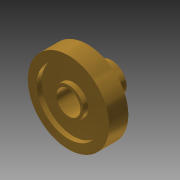
# Autodesk Inventor part: Spur Gear
Saved by Autodesk Inventor 2015 SP1 (Build 190203100, 203)
## iProperties
Created: 2015-02-24
Part Number: Spur Gear
Material: Brass, Soft Yellow
Document SubType Name: Modeling
Designer: Andrew
Density: 8.47 g/cm^3
Appearance: Brass - Satin
Author: Andrew
Autodesk Inventor part; units mm, degrees
ref_plane "YZ Plane" through (0, 0, 0) normal (1, 0, 0) x (0, 1, 0)
ref_plane "XZ Plane" through (0, 0, 0) normal (0, 1, 0) x (-1, 0, 0)
ref_plane "XY Plane" through (0, 0, 0) normal (0, 0, 1) x (1, 0, 0)
sketch "Sketch1" plane through (0, 0, 0) normal (0, 1, 0) x (-1, 0, 0)
  circle A0 centre (0, 0) radius 5
  circle A1 centre (0, 0) radius 10.5
  circle A2 centre (0, 0) radius 13.5
  line L0 (0, -18.9) -> (0, 18.9) projected
  line L1 (-18.9, 0) -> (18.9, 0) projected
  dimension "d0" = 10
  dimension "d1" = 21
  dimension "d2" = 27
  constraints: 3 centre point, 3 coincident
  measures "d0" diameter of A0
  measures "d1" diameter of A1
  measures "d2" diameter of A2
extrude "Extrusion1" add sketch "Sketch1" along normal mid plane 6.35 contours L1 A2 L0 A1 | A1 L0 A2 L1 | A1 L1 A2 L0 | L0 A2 L1 A1
extrude "Extrusion2" add sketch "Sketch1" along normal mid plane 3.175 contours L1 A1 L0 A0 | A0 L0 A1 L1 | A0 L1 A1 L0 | L0 A1 L1 A0
extrude "Extrusion3" add sketch "Sketch1" along normal mid plane 6.35 contours L1 L0 A0 | A0 L0 L1 | L0 L1 A0 | A0 L1 L0
sketch "Sketch2" plane through (0, 3.175, 0) normal (0, 1, 0) x (1, 0, 0)
  circle A0 centre (0, 0) radius 5 projected
extrude "Extrusion4" add sketch "Sketch2" along normal blind 7.9375
sketch "Sketch3" plane through (0, 11.1125, 0) normal (0, 1, 0) x (1, 0, 0)
  circle A0 centre (0, 0) radius 4
  dimension "d11" = 8
  constraints: 1 centre point, 1 coincident
  measures "d11" diameter of A0
extrude "Extrusion5" cut sketch "Sketch3" against normal up to next
sketch "Sketch4" plane through (0, 0, 0) normal (1, 0, 0) x (0, 1, 0)
  circle A0 centre (7.1437, 0) radius 1.5875
  line L0 (11.1125, 4) -> (11.1125, -4) projected
  line L1 (3.175, 10.5) -> (3.175, -10.5) projected
  line L2 (3.175, -13.5) -> (3.175, 13.5) construction
  line L3 (3.175, -4) -> (11.1125, -4) construction
  line L4 (11.1125, -4) -> (-3.175, -4) construction
  line L5 (7.1437, -4) -> (7.1437, 4) construction
  line L6 (11.1125, 4) -> (-3.175, 4) construction
  line L7 (-6.0325, 0) -> (13.97, 0) construction
  point P0 (0, 0)
  dimension "d14" = 3.175
  constraints: 4 end point, 3 point on line, 2 midpoint, 1 centre point, 1 collinear, 1 perpendicular
  measures "d14" diameter of A0
extrude "Extrusion6" cut sketch "Sketch4" along normal up to surface
body "Solid1"
